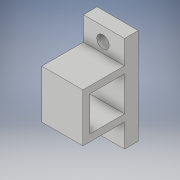
# Autodesk Inventor part: RailMountSupport
Saved by Autodesk Inventor 2019.3 (Build 233278000, 278)
## iProperties
Created: 2019-06-25
Part Number: RailMountSupport
Material: Generic
Document SubType Name: Modeling
Designer: mark
Density: 1 g/cm^3
Appearance: Default
Author: mark
Autodesk Inventor part; units mm, degrees
ref_plane "YZ Plane" through (0, 0, 0) normal (1, 0, 0) x (0, 1, 0)
ref_plane "XZ Plane" through (0, 0, 0) normal (0, 1, 0) x (-1, 0, 0)
ref_plane "XY Plane" through (0, 0, 0) normal (0, 0, 1) x (1, 0, 0)
ref_plane "Work Plane1" through (30, 2.888, 10) normal (0, 0, 1) x (1, 0, 0)
sketch "Sketch1" plane through (0, 0, 0) normal (0, 0, 1) x (1, 0, 0)
  circle A0 centre (-50, 10.188) radius 4.5
  circle A1 centre (-50, -39.812) radius 4.5
  line L0 (30, -49.812) -> (60, -49.812)
  line L1 (60, 20.188) -> (30, 20.188)
  line L2 (60, 2.888) -> (30, 2.888)
  line L3 (60, -32.512) -> (30, -32.512)
  line L4 (-64.29, 51.0493) -> (-64.29, -49.812)
  line L5 (-34.29, 20.188) -> (-64.29, 20.188)
  line L6 (-64.29, 20.188) -> (-64.29, -49.812)
  line L7 (-64.29, -49.812) -> (-34.29, -49.812)
  line L8 (-34.29, -49.812) -> (-34.29, 20.188)
  point P0 (0, 0)
extrude "Extrusion1" add sketch "Sketch1" along normal up to surface (10 mm away)
sketch "Sketch2" plane through (-64.29, -49.812, 0) normal (-1, 0, 0) x (0, 0, 1)
  line L0 (40.4, 52.7) -> (40.4, 17.3) projected
  line L1 (10, 52.7) -> (40.4, 52.7) projected
  line L2 (10, 17.3) -> (40.4, 17.3) projected
  line L3 (35.4, 22.3) -> (10, 22.3) projected
  line L4 (35.4, 22.3) -> (35.4, 47.7) projected
  line L5 (10, 47.7) -> (35.4, 47.7) projected
  line L6 (10, 0) -> (10, 70) projected
  point P0 (0, 49.812)
extrude "Extrusion2" add sketch "Sketch2" against normal up to surface (30 mm away) contours L0 L2 L6 L3 L4 L5 L1
body "Solid1"
